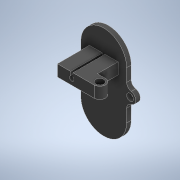
# Autodesk Inventor part: Base de la pinza 2
Saved by Autodesk Inventor 2021 (Build 250183000, 183)
## iProperties
Created: 2021-03-23
Part Number: Base de la pinza 2
Material: Generic
Document SubType Name: Modeling
Designer: LRC
Density: 1 g/cm^3
Appearance: Generic
Author: LRC
Autodesk Inventor part; units mm, degrees
ref_plane "YZ Plane" through (0, 0, 0) normal (1, 0, 0) x (0, 1, 0)
ref_plane "XZ Plane" through (0, 0, 0) normal (0, 1, 0) x (-1, 0, 0)
ref_plane "XY Plane" through (0, 0, 0) normal (0, 0, 1) x (1, 0, 0)
sketch "Sketch1" plane through (0, 0, 0) normal (0, 0, 1) x (1, 0, 0)
  line L0 (0, 10.45) -> (0, -10.45)
  arc A0 (10, 10.45) -> (-10, 10.45) centre (0, 10.45) ccw
  arc A1 (-10, -10.45) -> (10, -10.45) centre (0, -10.45) ccw
  line L1 (-10, 10.45) -> (-10, -10.45)
  line L2 (10, 10.45) -> (10, -10.45)
  point P0 (0, 0)
  point P1 (0, 0)
  dimension "d0" = 20.9
  dimension "d3" = 10
  dimension "d4" = 10
  constraints: 6 end point, 4 point on circle, 3 coincident, 2 centre point, 2 vertical, 1 midpoint, 1 parallel, 1 tangent
  measures "d0" distance of L0.start L0.end
  measures "d3" radius of A0
  measures "d4" radius of A1
extrude "Extrusion1" add sketch "Sketch1" along normal blind 2
sketch "Sketch2" plane through (0, 0, 2) normal (0, 0, 1) x (1, 0, 0)
  line L0 (-10, 10.45) -> (-10, -10.45) projected
  arc A0 (-10, -10.45) -> (10, -10.45) centre (0, -10.45) ccw projected
  line L1 (10, -10.45) -> (10, 10.45) projected
  arc A1 (10, 10.45) -> (-10, 10.45) centre (0, 10.45) ccw projected
  line L2 (-11.5, 0) -> (11.5, 0)
  circle A2 centre (-11.5, 0) radius 1.5
  circle A3 centre (11.5, 0) radius 1.5
  circle A4 centre (-11.5, 0) radius 2.5
  circle A5 centre (11.5, 0) radius 2.5
  point P0 (0, 0)
  point P1 (0, 0)
  dimension "d7" = 23
  dimension "d8" = 3
  dimension "d9" = 3
  dimension "d10" = 5
  dimension "d11" = 5
  constraints: 5 coincident, 4 centre point, 2 end point, 2 horizontal, 1 midpoint
  measures "d7" distance of L2.start L2.end
  measures "d8" diameter of A2
  measures "d9" diameter of A3
  measures "d10" diameter of A4
  measures "d11" diameter of A5
extrude "Extrusion2" add sketch "Sketch2" against normal blind 2 contours A4 L2 L0 | L0 A4 | L2 A4 L0 | A5 L1 | L1 L2 A5 | L2 L1 A5
fillet "Fillet1" radius 2.5 4 edges at (10, 2, 1) (10, -2, 1) (-10, 2, 1) (-10, -2, 1)
sketch "Sketch3" plane through (0, 0, 2) normal (0, 0, 1) x (1, 0, 0)
  circle A0 centre (11.5, 0) radius 1.5 projected
  arc A1 (12, -2.4495) -> (12, 2.4495) centre (11.5, 0) ccw projected
  arc A2 (10, 4.899) -> (12, 2.4495) centre (12.5, 4.899) ccw projected
  line L0 (10, 4.899) -> (10, 10.45) projected
  arc A3 (10, 10.45) -> (-10, 10.45) centre (0, 10.45) ccw
  line L1 (-10, 10.45) -> (-10, 4.899) projected
  arc A4 (-12, 2.4495) -> (-10, 4.899) centre (-12.5, 4.899) ccw projected
  arc A5 (-12, 2.4495) -> (-12, -2.4495) centre (-11.5, 0) ccw projected
  arc A6 (-10, -4.899) -> (-12, -2.4495) centre (-12.5, -4.899) ccw projected
  line L2 (-10, -4.899) -> (-10, -10.45) projected
  arc A7 (-10, -10.45) -> (10, -10.45) centre (0, -10.45) ccw projected
  line L3 (10, -10.45) -> (10, -4.899) projected
  arc A8 (12, -2.4495) -> (10, -4.899) centre (12.5, -4.899) ccw projected
  circle A9 centre (-11.5, 0) radius 1.5 projected
  line L4 (-6.25, 10.8) -> (-6.25, 5.8)
  line L5 (-6.25, 5.8) -> (6.25, 5.8)
  line L6 (6.25, 5.8) -> (6.25, 10.8)
  line L7 (11.5, 0) -> (0, 0)
  line L8 (0, 0) -> (5.75, 0)
  line L9 (-6.25, 10.8) -> (6.25, 10.8)
  point P0 (0, 0)
  point P1 (0, 10.45)
  dimension "d20" = 5.8
  dimension "d21" = 5
  dimension "d22" = 5
  constraints: 12 end point, 2 perpendicular, 2 point on circle, 1 centre point, 1 coincident, 1 horizontal, 1 midpoint, 1 vertical
  measures "d20" distance from line of L5 L8.end
  measures "d21" distance of L4.start L4.end
  measures "d22" distance of L5.end L6.end
extrude "Extrusion3" add sketch "Sketch3" along normal blind 14 contours L9 L6 L5 L4
sketch "Sketch4" plane through (0, 0, 16) normal (0, 0, 1) x (1, 0, 0)
  line L0 (-6.25, 5.8) -> (6.25, 5.8) projected
  line L1 (6.25, 5.8) -> (6.25, 10.8) projected
  line L2 (6.25, 10.8) -> (-6.25, 10.8) projected
  line L3 (-6.25, 10.8) -> (-6.25, 5.8) projected
  line L4 (-0.5, 10.8) -> (0.5, 10.8)
  line L5 (6.25, 10.8) -> (-6.25, 10.8) projected
  arc A0 (-0.5, 9.166) -> (0.5, 9.166) centre (0, 8.3) ccw
  line L6 (-0.5, 10.8) -> (-0.5, 9.166)
  line L7 (0.5, 10.8) -> (0.5, 9.166)
  point P0 (0, 0)
  point P1 (0, 10.8)
  point P2 (0, 10.8)
  dimension "d25" = 1
  dimension "d27" = 2
  constraints: 6 end point, 2 midpoint, 2 point on circle, 2 vertical, 1 centre point, 1 coincident, 1 horizontal
  measures "d25" distance of L4.start L4.end
  measures "d27" diameter of A0
extrude "Extrusion4" cut sketch "Sketch4" against normal blind 14 contours L2 L7 A0 L6
sketch "Sketch5" plane through (-6.25, 5.8, 2) normal (0, -1, 0) x (1, 0, 0)
  line L0 (12.5, 0) -> (0, 0) projected
  line L1 (12.5, 0) -> (12.5, 14) projected
  line L2 (0, 14) -> (12.5, 14) projected
  line L3 (0, 0) -> (0, 14) projected
  line L4 (12.5, 0) -> (12.5, 14) projected
  line L5 (12.5, 14) -> (16, 14)
  circle A0 centre (16, 11.5) radius 2.5
  circle A1 centre (16, 11.5) radius 1.75
  line L6 (16, 9) -> (12.5, 9)
  point P0 (6.25, -2)
  dimension "d30" = 3.5
  dimension "d33" = 3.5
  constraints: 4 end point, 2 horizontal, 1 centre point, 1 coincident, 1 point on line, 3 other
  measures "d30" distance of L1.end L5.end
  measures "d33" diameter of A1
extrude "Extrusion5" add sketch "Sketch5" against normal blind 5 contours L1 L5 A0 L6 | A0
body "Solid1"
